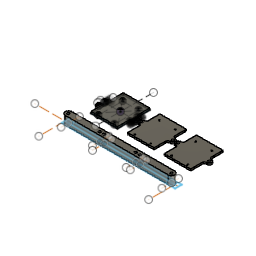
Multi FS40 Bracket v10 (Autodesk Fusion 360 design; units mm, degrees)
Autodesk Fusion 360 part; units mm, degrees
sketch "Schizzo1" plane through (0, 0, 0) normal (0, 0, 1) x (1, 0, 0)
  line L0 (32, -39) -> (-32, -39)
  line L1 (-32, -39) -> (-32, 39)
  line L2 (-32, 39) -> (32, 39)
  line L3 (32, 39) -> (32, -39)
  line L4 (32, -39) -> (-32, 39) construction
  line L5 (-32, -39) -> (32, 39) construction
  line L6 (-19.25, 24.7) -> (19.25, 24.7) construction
  line L7 (19.25, 24.7) -> (19.25, -33.8) construction
  line L8 (19.25, -33.8) -> (-19.25, -33.8) construction
  line L9 (-19.25, -33.8) -> (-19.25, 24.7) construction
  circle A0 centre (-19.25, 24.7) radius 1.7
  line L10 (0, 0) -> (0, 80) construction
  line L11 (0, 0) -> (0, -60) construction
  line L12 (-32, 0) -> (32, 0) construction
  circle A1 centre (-19.25, -33.8) radius 1.7
  circle A2 centre (19.25, -33.8) radius 1.7
  circle A3 centre (19.25, 24.7) radius 1.7
  line L13 (-32, 0) -> (-48, 0) construction
  line L14 (-38.2, 20.7498) -> (-38.2, -13.75) construction
  circle A4 centre (-38.2, 0) radius 6
  line L15 (-38.2, -6) -> (-46, -6) construction
  line L16 (-46, -9.1) -> (-32, -9.1) construction
  arc A5 (-32, -9.1) -> (-38.2, -6) centre (-38.2, -13.75) ccw
  arc A6 (-38.2, 6) -> (-32, 9.1) centre (-38.2, 13.75) ccw
  circle A7 centre (38.2, 0) radius 6
  arc A8 (32, 9.1) -> (38.2, 6) centre (38.2, 13.75) ccw
  arc A9 (38.2, -6) -> (32, -9.1) centre (38.2, -13.75) ccw
  line L17 (-47.0434, -78.6442) -> (226.9, -78.6442)
  line L18 (226.9, -78.6442) -> (226.9, -94.6442)
  line L19 (226.9, -94.6442) -> (-47.0434, -94.6442)
  line L20 (-47.0434, -94.6442) -> (-47.0434, -78.6442)
  circle A10 centre (-39.0434, -86.6442) radius 8
  line L21 (-39.0434, -60) -> (-39.0434, -104.1406) construction
  circle A11 centre (-39.0434, -86.6442) radius 2.9
  line L22 (37.3566, -65) -> (37.3566, -105) construction
  line L23 (226.9, -86.6442) -> (-120, -86.6442) construction
  circle A12 centre (37.3566, -86.6442) radius 2.9
  line L24 (47.4566, -68.4362) -> (47.4566, -114.7306) construction
  circle A13 centre (47.4566, -86.6442) radius 2.9
  line L25 (123.8566, -70) -> (123.8566, -110) construction
  circle A14 centre (123.8566, -86.6442) radius 2.9
  line L26 (133.9566, -70) -> (133.9566, -110) construction
  line L27 (210.3566, -70) -> (210.3566, -110) construction
  circle A15 centre (133.9566, -86.6442) radius 2.9
  circle A16 centre (210.3566, -86.6442) radius 2.9
  circle A17 centre (210.3566, -86.6442) radius 8
  line L28 (-47.0434, -86.6442) -> (218.3566, -86.6442)
  line L29 (218.3566, -86.6442) -> (-47.0434, -86.6442)
  line L30 (-47.0434, -86.6442) -> (-47.0434, -150) construction
  line L31 (218.3566, -86.6442) -> (218.3566, -150) construction
  circle A18 centre (-38.2, 0) radius 3.1
  circle A19 centre (38.2, 0) radius 3.1
  dimension "d1" = 64
  dimension "d2" = 78
  dimension "d3" = 33.8
  dimension "d5" = 58.5
  dimension "d6" = 19.25
  dimension "d7" = 38.5
  dimension "d8" = 3.4
  dimension "d9" = 3.4
  dimension "d17" = 6.2
  dimension "d18" = 12
  dimension "d19" = 3.1
  dimension "d20" = 76.4
  dimension "d21" = 16
  dimension "d22" = 8
  dimension "d23" = 5.8
  dimension "d24" = 76.4
  dimension "d25" = 5.8
  dimension "d28" = 86.5
  dimension "d29" = 5.8
  dimension "d30" = 76.4
  dimension "d32" = 5.8
  dimension "d33" = 86.5
  dimension "d34" = 76.4
  dimension "d35" = 5.8
  dimension "d36" = 5.8
  dimension "d39" = 6.2
  constraint horizontal L0
  constraint perpendicular L0 L1
  constraint parallel L0 L2
  constraint parallel L1 L3
  constraint coincident L4 L10.start
  constraint coincident L5 L10.start
  constraint coincident L10.start L11.start
  constraint horizontal L6
  constraint vertical L7
  constraint horizontal L8
  constraint vertical L9
  constraint coincident L6.start L9.end
  constraint perpendicular L2 L10
  constraint perpendicular L0 L11
  constraint midpoint L1 L12.start
  constraint midpoint L3 L12.end
  constraint coincident L8.end L9.start
  constraint symmetric A0 L11 A3
  constraint symmetric L11 A1 A2
  constraint perpendicular L1 L13
  constraint vertical L14
  constraint coincident A4 L15.start
  constraint coincident L14 L15.start
  constraint tangent A4 L15
  constraint horizontal L16
  constraint coincident L1 L16.end
  constraint coincident L14 A5.centre
  constraint symmetric L13 L15.start A6.start
  constraint symmetric L13 L16.end A6.end
  constraint symmetric L13 A5 A6
  constraint symmetric L10 A4 A7
  constraint symmetric L10 L15.start A9.start
  constraint symmetric L10 L16.end A9.end
  constraint symmetric L10 A5 A9
  constraint symmetric L10 A6.end A8.start
  constraint symmetric L10 A6.start A8.end
  constraint symmetric L10 A6 A8
  constraint horizontal L17
  constraint vertical L18
  constraint horizontal L19
  constraint vertical L20
  constraint tangent L20 A10
  constraint tangent L19 A10
  constraint perpendicular L17 L21
  constraint coincident A10.centre L21
  constraint concentric A10 A11
  constraint perpendicular L19 L22
  constraint midpoint L18 L23.start
  constraint perpendicular L21 L23
  constraint coincident L22 A12.centre
  constraint coincident L23 A12.centre
  constraint perpendicular L19 L24
  constraint coincident L24 A13.centre
  constraint coincident L23 A13.centre
  constraint perpendicular L19 L25
  constraint coincident L25 A14.centre
  constraint coincident L23 A14.centre
  constraint perpendicular L19 L26
  constraint perpendicular L19 L27
  constraint coincident L26 A15.centre
  constraint coincident L23 A15.centre
  constraint coincident L27 A16.centre
  constraint coincident L23 A16.centre
  constraint concentric A16 A17
  constraint tangent L17 A17
  constraint midpoint L20 L28.start
  constraint coincident A17 L28.end
  constraint coincident L23 L28.end
  constraint tangent A10 L30
  constraint perpendicular L28 L30
  constraint tangent A17 L31
  constraint coincident L14.end A5.centre
  constraint coincident L13 A4.centre
  constraint concentric A4 A18
  constraint symmetric L10 A18 A19
  measures "d1" distance of L1.end L2.end
  measures "d2" distance of L0.end L1.end
  measures "d3" distance of L10.start L8
  measures "d5" distance of L6 L8
  measures "d6" distance of L10.start L9
  measures "d7" distance of L7 L9
  measures "d8" diameter of A0
  measures "d9" diameter of A1
  measures "d17" distance of L1 L14.start
  measures "d18" diameter of A4
  measures "d19" distance of L15 L16
  measures "d20" distance of L14 A7.centre
  measures "d21" distance of L17.start L19.end
  measures "d22" radius of A10
  measures "d23" diameter of A11
  measures "d24" distance of L21 L22
  measures "d25" diameter of A12
  measures "d28" distance of A10.centre L24
  measures "d29" diameter of A13
  measures "d30" distance of L24 L25
  measures "d32" diameter of A14
  measures "d33" distance of L24 L26.end
  measures "d34" distance of L26 L27
  measures "d35" diameter of A15
  measures "d36" diameter of A16
  measures "d39" diameter of A18
extrude "Estrusione1" add sketch "Schizzo1" along normal blind 4 contours L0 L1 L2 L3 | L3 A7 A8 A9 | L1 A4 A5 A6 | A7 | A4 makes body 1
pattern_linear "Serie R1" count 1 spacing 0 along (0, 1, 0) count 3 spacing 88.5 along (1, 0, 0) of bodies 1 makes body 2 at (94.6333, 1.6759, 0) makes body 3 at (183.1333, 1.6759, 0)
extrude "Estrusione2" add sketch "Schizzo1" along normal blind 20 separate body contours L17 A10 A12 A13 A14 A15 A17 L28 L29 | A10 A11 L28 L29 | A10 A11 L28 L29 | A16 A17 L28 L29 | L19 A10 A12 A13 A14 A15 A17 L28 L29 | A16 A17 L28 L29 makes body 4
sketch "Schizzo2" plane through (0, 0, 0) normal (0, 0, 1) x (1, 0, 0)
  line L0 (-157.1405, -7.8769) -> (-137.1405, -7.8769)
  line L1 (-137.1405, -7.8769) -> (-137.1405, -4.8769)
  line L2 (-137.1405, -4.8769) -> (-157.1405, -4.8769)
  line L3 (-157.1405, -4.8769) -> (-157.1405, -7.8769)
  line L4 (-157.1405, -6.3769) -> (-137.1405, -6.3769) construction
  line L5 (-147.1405, -4.8769) -> (-147.1405, -7.8769) construction
  line L6 (-142.1405, -7.8769) -> (-152.1405, -7.8769)
  line L7 (-152.1405, -7.8769) -> (-152.1405, -4.8769)
  line L8 (-152.1405, -4.8769) -> (-142.1405, -4.8769)
  line L9 (-142.1405, -4.8769) -> (-142.1405, -7.8769)
  line L10 (-142.1405, -7.8769) -> (-152.1405, -4.8769) construction
  line L11 (-152.1405, -7.8769) -> (-142.1405, -4.8769) construction
  line L12 (-142.1405, -6.8769) -> (-152.1405, -6.8769)
  line L13 (-152.1405, -6.8769) -> (-152.1405, -5.8769)
  line L14 (-152.1405, -5.8769) -> (-142.1405, -5.8769)
  line L15 (-142.1405, -5.8769) -> (-142.1405, -6.8769)
  line L16 (-142.1405, -6.8769) -> (-152.1405, -5.8769) construction
  line L17 (-152.1405, -6.8769) -> (-142.1405, -5.8769) construction
  line L18 (-157.1405, 1.6231) -> (-47.1405, 1.6231)
  line L19 (-47.1405, 1.6231) -> (-47.1405, -14.3769)
  line L20 (-47.1405, -14.3769) -> (-157.1405, -14.3769)
  line L21 (-157.1405, -14.3769) -> (-157.1405, 1.6231)
  point P0 (-147.1405, -6.3769)
  point P1 (-147.1405, -6.3769)
  dimension "d40" = 20
  dimension "d41" = 3
  dimension "d42" = 10
  dimension "d43" = 3
  dimension "d44" = 10
  dimension "d45" = 1
  dimension "d50" = 110
  dimension "d51" = 8
  dimension "d52" = 16
  constraint horizontal L0
  constraint vertical L1
  constraint horizontal L2
  constraint vertical L3
  constraint midpoint L3 L4.start
  constraint midpoint L1 L4.end
  constraint midpoint L2 L5.start
  constraint midpoint L0 L5.end
  constraint horizontal L6
  constraint perpendicular L6 L7
  constraint parallel L6 L8
  constraint parallel L7 L9
  constraint coincident L10 P1
  constraint coincident L11 P1
  constraint midpoint L5 P1
  constraint horizontal L12
  constraint perpendicular L12 L13
  constraint parallel L12 L14
  constraint parallel L13 L15
  constraint coincident L16 P1
  constraint coincident L17 P1
  constraint coincident P1 P0
  constraint horizontal L18
  constraint vertical L19
  constraint horizontal L20
  constraint vertical L21
  constraint collinear L3 L21
  measures "d40" distance of L1 L3
  measures "d41" distance of L0 L2
  measures "d42" distance of L7.end L8.end
  measures "d43" distance of L6.end L7.end
  measures "d44" distance of L13.end L14.end
  measures "d45" distance of L12.end L13.end
  measures "d50" distance of L19 L21
  measures "d51" distance of L4.start L18.start
  measures "d52" distance of L18 L20
extrude "Estrusione3" add sketch "Schizzo2" along normal blind 4.5 separate body contours L0 L6 L7 L9 L12 | L2 L7 L8 L9 L14 makes body 5 at (-145.4738, -6.8769, 1.5) makes body 6 at (-145.4738, -4.8769, 1.5)
extrude "Estrusione4" add sketch "Schizzo2" against normal blind 20 separate body makes body 7
combine "Combina1" operation add target body 6 tool bodies 7
combine "Combina2" operation add target body 5 tool bodies 6
sketch "Schizzo3" plane through (-152.1405, 0, 0) normal (-1, 0, 0) x (0, -1, 0)
  line L0 (4.8769, 0) -> (5.8769, 0)
  line L1 (5.8769, 0) -> (5.8769, 4.5)
  line L2 (5.8769, 4.5) -> (4.8769, 4.5)
  line L3 (4.8769, 4.5) -> (4.8769, 0)
sketch "Schizzo5" plane through (-152.1405, -5.3769, 2.25) normal (-1, 0, 0) x (0, -1, 0)
  line L0 (0.5, 2.25) -> (0.5, 4.484) construction
  line L1 (1.5, 2.25) -> (1.5, 4.4786) construction
  line L2 (0.5, 2.25) -> (1.5, 2.25) construction
  line L3 (1, 2.25) -> (1, 4.5) construction
  line L4 (0.5, 2.25) -> (-2.3514, 2.25) construction
  line L5 (0.5, 2.25) -> (-1, 2.25)
  line L6 (0.5, 2.25) -> (0.5, 4.25)
  line L7 (0.5, 4.25) -> (-1, 2.25)
  line L8 (1.5, 4.25) -> (3, 2.25)
  line L9 (1.5, 2.25) -> (3, 2.25)
  line L10 (1.5, 2.25) -> (1.5, 4.25)
  dimension "d59" = 1.5
  dimension "d60" = 2
  constraint vertical L0
  constraint vertical L1
  constraint midpoint L2 L3.start
  constraint perpendicular L2 L3
  constraint perpendicular L0 L4
  constraint perpendicular L0 L5
  constraint coincident L0 L6.end
  constraint symmetric L0.start L3 L1.start
  constraint symmetric L3 L5.end L8.end
  constraint symmetric L3 L6.end L8.start
  measures "d59" distance of L0.start L5.end
  measures "d60" distance of L2 L6.end
extrude "Estrusione6" add sketch "Schizzo5" against normal blind 10 bodies 5
hidden bodies 5
equation "d6 = 38.50 mm / 2"
named bodies: "Basetta 1", "Basetta 2", "Basetta 3", "Trave", "Fissaggio Lampada"
